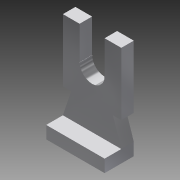
# Autodesk Inventor part: Guide Fork CAD
Saved by Autodesk Inventor 2015 (Build 190159000, 159)
## iProperties
Created: 2015-01-16
Part Number: Guide Fork CAD
Material: Aluminum 6061
Document SubType Name: Modeling
Designer: 201132652
Density: 2.7 g/cm^3
Appearance: Aluminum - Polished
Author: 201132652
Autodesk Inventor part; units mm, degrees
ref_plane "YZ Plane" through (0, 0, 0) normal (1, 0, 0) x (0, 1, 0)
ref_plane "XZ Plane" through (0, 0, 0) normal (0, 1, 0) x (-1, 0, 0)
ref_plane "XY Plane" through (0, 0, 0) normal (0, 0, 1) x (1, 0, 0)
sketch "Sketch1" plane through (0, 0, 0) normal (0, 0, 1) x (1, 0, 0)
  line L0 (0, 0) -> (88.9, 0)
  line L1 (88.9, 0) -> (88.9, 152.4)
  line L2 (88.9, 152.4) -> (0, 152.4)
  line L3 (0, 152.4) -> (0, 0)
  dimension "d0" = 152.4
  dimension "d1" = 88.9
  constraints: 8 end point, 2 parallel, 1 horizontal, 1 perpendicular
  measures "d0" distance of L2.end L0.start
  measures "d1" distance of L0.start L0.end
extrude "Extrusion1" add sketch "Sketch1" along normal blind 19.05
sketch "Sketch2" plane through (0, 0, 19.05) normal (0, 0, 1) x (1, 0, 0)
  line L0 (0, 0) -> (88.9, 0)
  line L1 (88.9, 0) -> (88.9, 19.05)
  line L2 (88.9, 19.05) -> (0, 19.05)
  line L3 (0, 19.05) -> (0, 0)
  line L4 (88.9, 0) -> (88.9, 152.4) projected
  dimension "d4" = 19.05
  constraints: 8 end point, 2 parallel, 1 collinear, 1 horizontal, 1 perpendicular
  measures "d4" distance of L0.end L1.end
extrude "Extrusion2" add sketch "Sketch2" along normal blind 25.4
sketch "Sketch3" plane through (0, 0, 19.05) normal (0, 0, 1) x (1, 0, 0)
  line L0 (25.4, 166.2997) -> (63.5, 166.2997)
  line L1 (63.5, 166.2997) -> (63.5, 101.6)
  line L2 (63.5, 101.6) -> (25.4, 101.6)
  line L3 (25.4, 101.6) -> (25.4, 166.2997)
  line L4 (88.9, 152.4) -> (0, 152.4) projected
  arc A0 (25.6076, 101.6) -> (63.2924, 101.6) centre (44.45, 101.6) ccw
  point P0 (0, 0)
  dimension "d7" = 25.4
  dimension "d8" = 25.4
  dimension "d9" = 50.8
  constraints: 8 end point, 2 parallel, 2 perpendicular, 2 point on circle, 2 point on line, 1 centre point, 1 horizontal, 1 midpoint
  measures "d7" distance from line of L1 L4.start
  measures "d8" distance from line of L3 L4.end
  measures "d9" distance from line of L2.end L4
extrude "Extrusion3" cut sketch "Sketch3" against normal blind 25.4
sketch "Sketch4" plane through (0, 0, 19.05) normal (0, 0, 1) x (1, 0, 0)
  line L0 (0, 19.05) -> (12.7, 57.15)
  line L1 (12.7, 57.15) -> (0, 57.15)
  line L2 (0, 19.05) -> (88.9, 19.05) projected
  line L3 (0, 19.05) -> (0, 57.15)
  line L4 (0, 152.4) -> (0, 0) projected
  line L5 (88.9, 19.05) -> (88.9, 57.15)
  line L6 (88.9, 0) -> (88.9, 152.4) projected
  line L7 (76.2, 57.15) -> (88.9, 19.05)
  line L8 (76.2, 57.15) -> (88.9, 57.15)
  line L9 (88.9, 19.05) -> (88.9, 57.15)
  dimension "d12" = 12.7
  dimension "d13" = 38.1
  dimension "d14" = 12.7
  dimension "d15" = 38.1
  constraints: 14 end point, 2 perpendicular, 2 point on line, 1 parallel
  measures "d12" distance of L0.end L1.end
  measures "d13" distance of L0.start L1.end
  measures "d14" distance of L7.start L5.end
  measures "d15" distance of L2.end L5.end
extrude "Extrusion4" cut sketch "Sketch4" against normal blind 25.4 contours L3 L1 L0
sketch "Sketch5" plane through (0, 0, 19.05) normal (0, 0, 1) x (1, 0, 0)
  line L0 (88.9, 19.05) -> (76.2, 57.15)
  line L1 (76.2, 57.15) -> (88.9, 57.15)
  line L2 (88.9, 19.05) -> (88.9, 152.4) projected
  point P0 (0, 0)
  dimension "d18" = 12.7
  dimension "d19" = 38.1
  constraints: 4 end point, 1 horizontal, 1 point on line
  measures "d18" distance of L0.end L1.end
  measures "d19" distance of L0.start L1.end
extrude "Extrusion5" cut sketch "Sketch5" against normal blind 25.4
body "Solid1"
